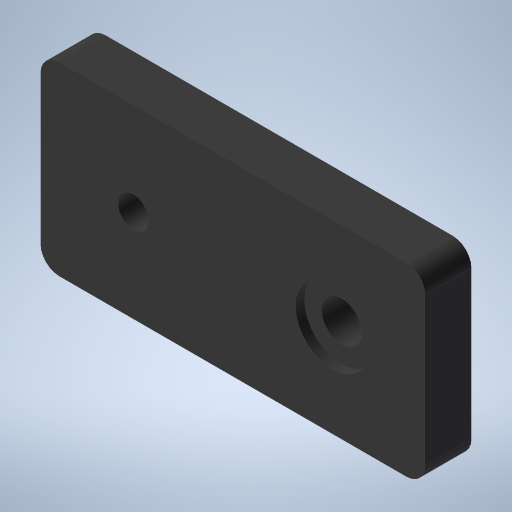
# Autodesk Inventor part: PSU_bracket
Saved by Autodesk Inventor 2024.2 (Build 282272000, 272)
## iProperties
Created: 2024-06-02
Part Number: PSU_bracket
Material: Generic
Document SubType Name: Modeling
Designer: Micha
Density: 1 g/cm^3
Appearance: Default
Author: Micha
Autodesk Inventor part; units mm, degrees
ref_plane "YZ Plane" through (0, 0, 0) normal (1, 0, 0) x (0, 1, 0)
ref_plane "XZ Plane" through (0, 0, 0) normal (0, 1, 0) x (-1, 0, 0)
ref_plane "XY Plane" through (0, 0, 0) normal (0, 0, 1) x (1, 0, 0)
sketch "Sketch1" plane through (0, 0, 0) normal (0, 0, 1) x (1, 0, 0)
  line L0 (0, 0) -> (41.5, 0)
  line L1 (41.5, 0) -> (41.5, 20)
  line L2 (41.5, 20) -> (0, 20)
  line L3 (0, 20) -> (0, 0)
  circle A0 centre (31.5, 10) radius 2.175
  circle A1 centre (10, 10) radius 1.675
  line L4 (20, 20) -> (20, 0) construction
  point P0 (41.5, 10)
  dimension "d0" = 41.5
  dimension "d1" = 4.35
  dimension "d2" = 3.35
  dimension "d3" = 20
  dimension "d4" = 10
  dimension "d5" = 10
  dimension "d6" = 11.5
  constraints: 10 end point, 2 centre point, 2 horizontal alignment, 2 parallel, 2 perpendicular, 2 point on line, 1 horizontal, 1 midpoint
  measures "d0" distance of L1.end L2.end
  measures "d1" diameter of A0
  measures "d2" diameter of A1
  measures "d3" distance of L0.end L1.end
  measures "d4" distance from line of L3 A1.centre
  measures "d5" distance from line of L4 A1.centre
  measures "d6" distance from line of L4 A0.centre
extrude "Extrusion1" add sketch "Sketch1" along normal blind 5
sketch "Sketch2" plane through (0, 0, 5) normal (0, 0, 1) x (1, 0, 0)
  circle A0 centre (31.5, 10) radius 2.175 projected
  circle A1 centre (31.5, 10) radius 4
  point P0 (0, 0)
  dimension "d9" = 8
  constraints: 1 centre point, 1 coincident
  measures "d9" diameter of A1
extrude "Extrusion2" cut sketch "Sketch2" against normal blind 1
fillet "Fillet1" radius 2 4 edges at (0, 20, 2.5) (41.5, 20, 2.5) (41.5, 0, 2.5) (0, 0, 2.5)
body "Solid1"
